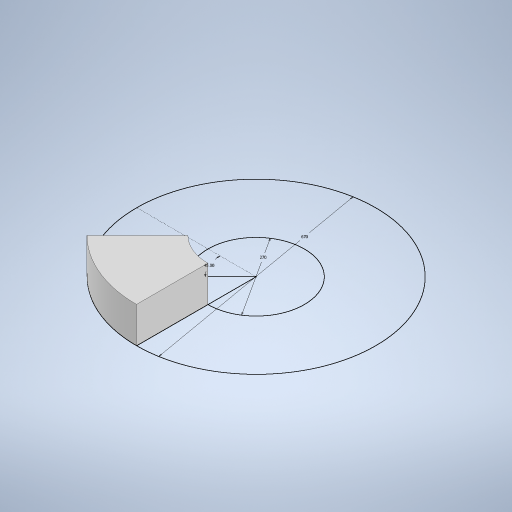
# Autodesk Inventor part: Test
Saved by Autodesk Inventor 2023 (Build 270158000, 158)
## iProperties
Created: 2022-11-13
Part Number: Test
Material: Generic
Document SubType Name: Modeling
Designer: mihal
Density: 1 g/cm^3
Appearance: Default
Author: mihal
Autodesk Inventor part; units mm, degrees
ref_plane "YZ Plane" through (0, 0, 0) normal (1, 0, 0) x (0, 1, 0)
ref_plane "XZ Plane" through (0, 0, 0) normal (0, 1, 0) x (-1, 0, 0)
ref_plane "XY Plane" through (0, 0, 0) normal (0, 0, 1) x (1, 0, 0)
sketch "Sketch1" plane through (0, 0, 0) normal (0, 1, 0) x (-1, 0, 0)
  circle A0 centre (0, 0) radius 135
  circle A1 centre (0, 0) radius 335
  line L0 (0, 0) -> (0, 335)
  line L1 (0, 0) -> (236.8808, 236.8808)
  line L2 (0, 0) -> (335, 0) construction
  point P0 (95.4594, 95.4594)
  point P1 (0, 135)
  dimension "d0" = 270
  dimension "d1" = 670
  dimension "d2" = 45
  constraints: 6 end point, 2 centre point, 2 coincident, 2 point on circle, 1 equal length, 1 horizontal, 1 vertical
  measures "d0" diameter of A0
  measures "d1" diameter of A1
  measures "d2" angle of L2 L1
extrude "Extrusion1" add sketch "Sketch1" along normal blind 100 contours A0 L0 A1 L1 picked at (100.2741, 248.6764)
body "Solid1"
